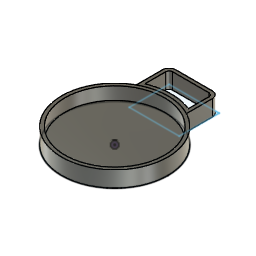
firstDraft_circularShell (Autodesk Fusion 360 design; units mm, degrees)
part number: 2025-07-12-21-23-09-506
Autodesk Fusion 360 part; units mm, degrees
note: some values were not read from the file. Set by a fixed rule: which face or edge a step refers to.
sketch "Sketch2" plane through (0, 0, 0) normal (0, 0, 1) x (1, 0, 0)
  circle A0 centre (0, 0) radius 40
  line L0 (-19, 60) -> (18.612, 60)
  line L1 (18.612, 60) -> (18.612, 30)
  line L2 (18.612, 30) -> (-19, 30)
  line L3 (-19, 30) -> (-19, 60)
  dimension "d6" = 80
  dimension "d12" = 30
  constraint coincident A0.centre origin
  constraint horizontal L0
  constraint vertical L1
  constraint horizontal L2
  constraint vertical L3
  measures "d6" diameter of A0
  measures "d12" distance of L0.start L2.end
extrude "Extrude1" add sketch "Sketch2" along normal blind 12 contours A0 L1 L2 L3 | A0 L1 L2 L3 makes body 1
shell "Shell1" thickness 2.5 removed faces 1 at (11.5919, 10.121, 12) on bodies 1
sketch "Sketch3" plane through (0, 0, 2.5) normal (0, 0, 1) x (-1, 0, 0)
  circle A0 centre (0, 0) radius 37.5
extrude "Extrude2" add sketch "Sketch2" along normal blind 12 separate body contours A0 L0 L1 L3 makes body 2
fillet "Fillet1" radius 5 2 edges at (-19, 60, 6) (18.612, 60, 6) on bodies 2
shell "Shell2" thickness 2.5 removed faces 1 at (0.7291, 53.3057, 12) on bodies 2
extrude "Extrude3" cut 1 faces at (-0.1993, 52.4998, 2.5) along direction (0, 0, -1) blind 5 on bodies 2 bodies 2
sketch "Sketch1" plane through (0, 0, 0) normal (0, 0, 1) x (1, 0, 0)
equation "diameter = 80 mm"
equation "shell = 2.5 mm"
equation "height = 12 mm"
equation "gap = 0.2 mm"
equation "d6 = diameter"
equation "d7 = height"
equation "d9 = shell"
equation "extend_width = 30 mm"
equation "extend_height = 30 mm"
equation "d12 = extend_height"
equation "d13 = height"
equation "d17 = shell"
